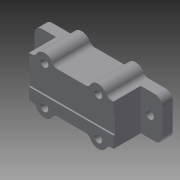
# Autodesk Inventor part: y-belt-holder
Saved by Autodesk Inventor 2015 (Build 190159000, 159)
## iProperties
Created: 2015-04-29
Part Number: y-belt-holder
Material: Generic
Document SubType Name: Modeling
Designer: X
Density: 1 g/cm^3
Appearance: Default
Author: X
Autodesk Inventor part; units mm, degrees
ref_plane "YZ Plane" through (0, 0, 0) normal (1, 0, 0) x (0, 1, 0)
ref_plane "XZ Plane" through (0, 0, 0) normal (0, 1, 0) x (-1, 0, 0)
ref_plane "XY Plane" through (0, 0, 0) normal (0, 0, 1) x (1, 0, 0)
sketch "Sketch1" plane through (0, 0, 0) normal (0, 1, 0) x (-1, 0, 0)
  line L0 (-25, 8) -> (25, 8)
  line L1 (25, 8) -> (25, -8)
  line L2 (25, -8) -> (-25, -8)
  line L3 (-25, -8) -> (-25, 8)
  line L4 (-25, 8) -> (25, -8) construction
  line L5 (25, 8) -> (-25, -8) construction
  circle A0 centre (10.5, 7.5) radius 3.5
  circle A1 centre (-10.5, 7.5) radius 3.5
  circle A2 centre (10.5, -7.5) radius 3.5
  circle A3 centre (-10.5, -7.5) radius 3.5
  line L6 (10.5, 7.5) -> (10.5, -7.5) construction
  line L7 (10.5, -7.5) -> (-10.5, -7.5) construction
  line L8 (-10.5, -7.5) -> (-10.5, 7.5) construction
  line L9 (-10.5, 7.5) -> (10.5, 7.5) construction
  line L10 (10.5, 7.5) -> (-10.5, -7.5) construction
  line L11 (-10.5, 7.5) -> (10.5, -7.5) construction
  point P0 (0, 0)
  point P1 (0, 0)
  point P2 (0, 0)
  dimension "d0" = 16
  dimension "d1" = 50
  dimension "d4" = 21
  dimension "d5" = 7
  dimension "d31" = 15
  constraints: 24 end point, 5 midpoint, 4 centre point, 4 coincident, 4 perpendicular, 3 equal radius, 3 parallel, 1 horizontal
  measures "d0" distance of L0.end L1.end
  measures "d1" distance of L0.start L0.end
  measures "d4" distance of L8.end L6.start
  measures "d5" diameter of A0
  measures "d31" distance between parallel lines of L7 L9
extrude "Extrusion2" add sketch "Sketch1" along normal blind 14.6
sketch "Sketch2" plane through (0, 0, 0) normal (0, -1, 0) x (1, 0, 0)
  line L0 (-25, 8) -> (-16.5, 8)
  line L1 (-16.5, 8) -> (-16.5, -8)
  line L2 (-16.5, -8) -> (-25, -8)
  line L3 (-25, -8) -> (-25, 8)
  line L4 (0, 8) -> (0, -8) construction
  line L5 (7.0359, -8) -> (-7.0359, -8) construction
  line L6 (-25, -8) -> (-13.9641, -8) construction
  line L7 (25, 8) -> (16.5, 8)
  line L8 (16.5, 8) -> (16.5, -8)
  line L9 (16.5, -8) -> (25, -8)
  line L10 (25, -8) -> (25, 8)
  point P0 (0, 0)
  dimension "d8" = 8.5
  constraints: 18 end point, 4 symmetric about line, 2 midpoint, 2 parallel, 1 collinear, 1 horizontal, 1 perpendicular, 1 vertical
  measures "d8" distance of L0.start L0.end
extrude "Extrusion3" cut sketch "Sketch2" against normal blind 10.6
sketch "Sketch3" plane through (0, 0, 0) normal (0, -1, 0) x (1, 0, 0)
  line L0 (-7.0359, 8) -> (7.0359, 8) construction
  line L1 (0, 8) -> (0, -7.6173) construction
  line L2 (-25, -8) -> (-25, 8) construction
  line L3 (-25, 0) -> (25, 0) construction
  line L4 (25, 8) -> (25, -8) construction
  point P0 (0, 0)
  point P1 (-20, 0)
  point P2 (20, 0)
  dimension "d12" = 20
  constraints: 4 end point, 3 midpoint, 1 point on line, 1 symmetric about line, 1 vertical
  measures "d12" distance from line of L1 point (-20, 0)
hole "Hole1" at (-20, 0, 0) at (20, 0, 0) direction (0, 1, 0) diameter 3.2 end through all
hole "Hole2" at (-10.5, 0, 7.5) at (10.5, 0, 7.5) at (10.5, 0, -7.5) at (-10.5, 0, -7.5) direction (0, 1, 0) diameter 2.4 end through all countersink diameter 3 countersink angle 45
fillet "Fillet1" radius 2 8 edges at (-7.0359, 7.3, 8) (-13.9641, 7.3, 8) (13.9641, 7.3, 8) (7.0359, 7.3, 8) (13.9641, 7.3, -8) (7.0359, 7.3, -8) (-7.0359, 7.3, -8) (-13.9641, 7.3, -8)
fillet "Fillet2" radius 3 4 edges at (-25, 12.6, 8) (-25, 12.6, -8) (25, 12.6, 8) (25, 12.6, -8)
sketch "Sketch4" plane through (0, 0, 0) normal (0, -1, 0) x (1, 0, 0)
  line L0 (16.5, -8) -> (16.5, 8) projected
  line L1 (-16.5, -3.5) -> (16.5, -3.5)
  line L2 (16.5, -3.5) -> (16.5, 3.5)
  line L3 (16.5, 3.5) -> (-16.5, 3.5)
  line L4 (-16.5, 3.5) -> (-16.5, -3.5)
  line L5 (-16.5, -3.5) -> (16.5, 3.5) construction
  line L6 (16.5, -3.5) -> (-16.5, 3.5) construction
  point P0 (0, 0)
  dimension "d32" = 7
  constraints: 12 end point, 2 midpoint, 2 parallel, 1 horizontal, 1 perpendicular, 1 point on line
  measures "d32" distance between parallel lines of L1 L3
extrude "Extrusion4" cut sketch "Sketch4" against normal blind 0.6
body "Solid2"
